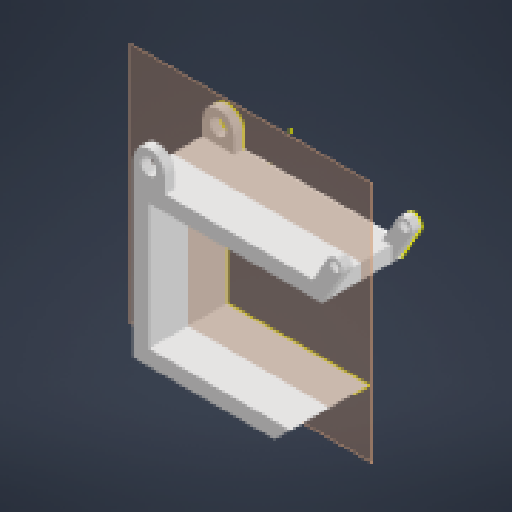
# Autodesk Inventor part: Claw New
Saved by Autodesk Inventor 2023.6 (Build 276521000, 521)
## iProperties
Created: 2026-03-04
Part Number: Claw New
Material: Generic
Document SubType Name: Modeling
Designer: user
Density: 1 g/cm^3
Appearance: Default
Author: user
Autodesk Inventor part; units mm, degrees
ref_plane "YZ Plane" through (0, 0, 0) normal (1, 0, 0) x (0, 1, 0)
ref_plane "XZ Plane" through (0, 0, 0) normal (0, 1, 0) x (-1, 0, 0)
ref_plane "XY Plane" through (0, 0, 0) normal (0, 0, 1) x (1, 0, 0)
sketch "Sketch1" plane through (0, 0, 0) normal (0, 0, 1) x (1, 0, 0)
  circle A0 centre (-20.2579, 7.5645) radius 2.5
  line L0 (34.7421, -2.4355) -> (34.7421, 2.5645)
  line L1 (34.7421, 2.5645) -> (-15.2579, 2.5645)
  line L2 (-15.2579, 2.5645) -> (-15.2579, 7.5645)
  arc A1 (-15.2579, 7.5645) -> (-25.2579, 7.5645) centre (-20.2579, 7.5645) ccw
  line L3 (-25.2579, 7.5645) -> (-25.2579, -62.4355)
  line L4 (-25.2579, -62.4355) -> (4.7421, -62.4355)
  line L5 (9.7421, -57.4355) -> (4.7421, -62.4355)
  line L6 (-20.2579, -57.4355) -> (9.7421, -57.4355)
  line L7 (-20.2579, -2.4355) -> (-20.2579, -57.4355)
  line L8 (-20.2579, -2.4355) -> (34.7421, -2.4355)
  line L9 (-15.2579, 2.5645) -> (-25.2579, 2.5645)
  point P0 (0, 0)
  point P1 (4.7421, 37.5645)
  dimension "d0" = 5
  dimension "d1" = 5
  dimension "d2" = 30
  dimension "d3" = 55
  dimension "d4" = 5
  dimension "d5" = 5
  dimension "d6" = 5
  dimension "d7" = 65
  dimension "d8" = 5
  dimension "d24" = 30
  constraints: 20 end point, 2 centre point, 2 point on circle, 1 coincident, 1 perpendicular, 1 point on line
  measures "d0" distance between parallel lines of L7 L3
  measures "d1" distance between parallel lines of L4 L6
  measures "d2" distance of L6.start L5.start
  measures "d3" distance between parallel lines of L7 L0
  measures "d4" distance between parallel lines of L8 L1
  measures "d5" diameter of A0
  measures "d6" radius of A1
  measures "d7" distance between parallel lines of L4 L9
  measures "d8" distance of L1.end L2.end
  measures "d24" distance of L3.end L4.end
extrude "Extrusion1" add sketch "Sketch1" along normal blind 25
ref_plane "Work Plane1" through (0, 0, 12.5) normal (0, 0, 1) x (1, 0, 0)
sketch "Sketch2" plane through (0, 0, 12.5) normal (0, 0, 1) x (1, 0, 0)
  line L0 (-15.2579, 2.5645) -> (-15.2579, 7.5645) projected
  line L1 (34.7421, 2.5645) -> (-15.2579, 2.5645) projected
  line L2 (34.7421, -2.4355) -> (34.7421, 2.5645) projected
  line L3 (-20.2579, -2.4355) -> (34.7421, -2.4355) projected
  line L4 (-20.2579, -57.4355) -> (-20.2579, -2.4355) projected
  line L5 (9.7421, -57.4355) -> (-20.2579, -57.4355) projected
  line L6 (4.7421, -62.4355) -> (9.7421, -57.4355) projected
  line L7 (-25.2579, -62.4355) -> (4.7421, -62.4355) projected
  line L8 (-25.2579, 7.5645) -> (-25.2579, -62.4355) projected
  arc A0 (-15.2579, 7.5645) -> (-25.2579, 7.5645) centre (-20.2579, 7.5645) ccw projected
  circle A1 centre (-20.2579, 7.5645) radius 2.5 projected
  line L9 (-15.2579, 2.5645) -> (-15.2579, 7.5645) projected
  line L10 (-15.2579, 2.5645) -> (-25.2579, 2.5645)
  line L11 (-25.2579, 7.5645) -> (-25.2579, -62.4355) projected
  point P0 (0, 0)
  constraints: 2 end point, 1 perpendicular, 1 point on line
extrude "Extrusion2" cut sketch "Sketch2" along normal mid plane 19 contours L10 L8 A0 L0
sketch "Sketch3" plane through (0, 0, 12.5) normal (0, 0, 1) x (1, 0, 0)
  line L0 (-20.2579, -2.4355) -> (34.7421, -2.4355) projected
  line L1 (34.7421, -2.4355) -> (42.2421, 10.5548)
  line L2 (34.7421, -2.4355) -> (34.7421, 2.5645) projected
  line L3 (34.7421, 2.5645) -> (40.0771, 11.8048)
  circle A0 centre (38.8271, 9.6398) radius 1.5
  line L4 (34.7421, 2.5645) -> (-15.2579, 2.5645) projected
  line L5 (42.2421, 10.5548) -> (40.0771, 11.8048)
  line L6 (40.0771, 11.8048) -> (37.912, 13.0548)
  line L7 (37.912, 13.0548) -> (31.8554, 2.5645)
  circle A1 centre (38.8271, 9.6398) radius 2.5
  point P0 (0, 0)
  point P1 (36.662, 10.8898)
  point P2 (40.9921, 8.3898)
  dimension "d13" = 15
  dimension "d14" = 30
  dimension "d15" = 3
  dimension "d16" = 2.5
  dimension "d17" = 60
  dimension "d18" = 2.5
  dimension "d19" = 2.5
  constraints: 10 end point, 3 point on line, 2 centre point, 2 tangent, 1 coincident, 1 perpendicular
  measures "d13" distance of L0.end L1.end
  measures "d14" angle of L2 L1
  measures "d15" diameter of A0
  measures "d16" distance between parallel lines of L1 L3
  measures "d17" angle of L4 L3
  measures "d18" distance of L3.end L6.end
  measures "d19" distance between parallel lines of L3 L7
extrude "Extrusion3" add sketch "Sketch3" along normal mid plane 25 contours L2 L3 A1 L1 | A1 L3 A0 | L4 L7 A1 L3 | A1 L3 A0
extrude "Extrusion4" cut sketch "Sketch3" along normal mid plane 19 contours L2 L3 A1 L1 | A1 L3 A0 | L4 L7 A1 L3 | A1 L3 A0
sketch "Sketch4" plane through (0, 0, 0) normal (0, 0, -1) x (-1, 0, 0)
  circle A0 centre (-38.8271, 9.6398) radius 1.5 projected
  line L0 (15.2579, 2.5645) -> (15.2579, 7.5645) projected
  line L1 (-31.8554, 2.5645) -> (15.2579, 2.5645) projected
  line L2 (-31.8554, 2.5645) -> (-36.662, 10.8898) projected
  arc A1 (-36.662, 10.8898) -> (-40.9921, 8.3898) centre (-38.8271, 9.6398) ccw projected
  line L3 (-40.9921, 8.3898) -> (-34.7421, -2.4355) projected
  line L4 (20.2579, -2.4355) -> (-34.7421, -2.4355) projected
  line L5 (20.2579, -57.4355) -> (20.2579, -2.4355) projected
  line L6 (-9.7421, -57.4355) -> (20.2579, -57.4355) projected
  line L7 (-4.7421, -62.4355) -> (-9.7421, -57.4355) projected
  line L8 (25.2579, -62.4355) -> (-4.7421, -62.4355) projected
  line L9 (25.2579, 7.5645) -> (25.2579, -62.4355) projected
  arc A2 (25.2579, 7.5645) -> (15.2579, 7.5645) centre (20.2579, 7.5645) ccw projected
  circle A3 centre (20.2579, 7.5645) radius 2.5 projected
  line L10 (20.2579, -2.4355) -> (-34.7421, -2.4355) projected
  line L11 (-31.8554, 2.5645) -> (-34.7421, 2.5645) projected
  line L12 (-34.7421, -2.4355) -> (-34.7421, 2.5645)
  line L13 (-34.7421, 2.5645) -> (-31.8554, 2.5645)
  line L14 (-31.8554, 2.5645) -> (25.2579, 2.5645)
  line L15 (25.2579, 7.5645) -> (25.2579, -62.4355) projected
  point P0 (0, 0)
  constraints: 6 end point, 2 point on line, 1 perpendicular, 1 vertical
body "Solid1"
